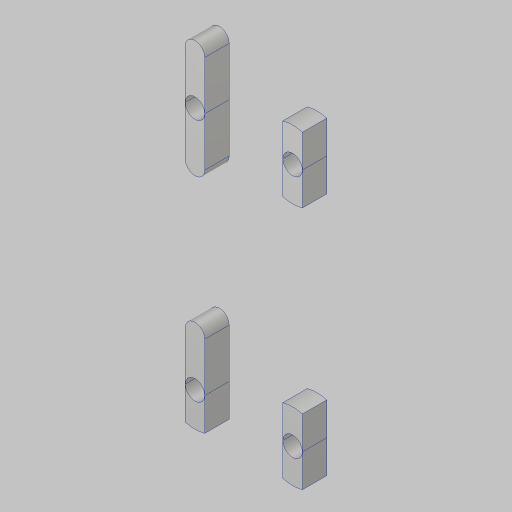
# Autodesk Inventor part: CL8-GB-001
Saved by Autodesk Inventor 2023.5 (Build 275446000, 446)
## iProperties
Created: 2025-03-18
Part Number: CL8-GB-001
Material: Aluminum 6061
Document SubType Name: Modeling
Designer: slick
Density: 2.7 g/cm^3
Appearance: Aluminum - Flat
Mass: 157.99 g
Surface Area: 311.753 cm^2
Volume: 58.5147 cm^3
Author: slick
Autodesk Inventor part; units mm, degrees
ref_plane "YZ Plane" through (0, 0, 0) normal (1, 0, 0) x (0, 1, 0)
ref_plane "XZ Plane" through (0, 0, 0) normal (0, 1, 0) x (-1, 0, 0)
ref_plane "XY Plane" through (0, 0, 0) normal (0, 0, 1) x (1, 0, 0)
sketch "Sketch1" plane through (0, 0, 0) normal (0, 0, 1) x (1, 0, 0)
  line L0 (0, 0) -> (-50.8, 0) construction
  line L1 (-50.8, 0) -> (-50.8, 381) construction
  line L2 (-50.8, 381) -> (0, 381) construction
  line L3 (0, 381) -> (0, 0) construction
  circle A0 centre (-50.8, 431.8) radius 11.1125 construction
  line L4 (-50.8, 353.7099) -> (-298.4703, 0) construction
  line L5 (-298.4703, 0) -> (-267.4626, 0) construction
  line L6 (-267.4626, 0) -> (-50.8, 309.4263) construction
  dimension "d0" = 50.8
  dimension "d1" = 381
  dimension "d2" = 22.225
  dimension "d3" = 431.8
  dimension "d4" = 50.8
  dimension "d5" = 431.8
  dimension "d6" = 25.4
  dimension "d7" = 35
  constraints: 14 end point, 3 parallel, 2 horizontal, 2 point on line, 1 centre point, 1 collinear, 1 perpendicular
  measures "d0" distance of L1.end L2.end
  measures "d1" distance of L0.end L1.end
  measures "d2" diameter of A0
  measures "d3" distance from line of L0 A0.centre
  measures "d4" distance from line of L3 A0.centre
  measures "d5" distance of L4.start L4.end
  measures "d6" distance between parallel lines of L6 L4
  measures "d7" angle of L1 L4
sketch "Sketch2" plane through (0, 0, 0) normal (0, 0, 1) x (1, 0, 0)
  line L0 (-267.4626, 0) -> (-50.8, 309.4263) construction
  line L1 (-50.8, 353.7099) -> (-298.4703, 0) construction
  line L2 (-50.8, 0) -> (-50.8, 381) construction
  line L3 (0, 381) -> (0, 0) construction
  line L4 (-50.8, 381) -> (0, 381) construction
  circle A0 centre (-50.8, 431.8) radius 11.1125 construction
  line L5 (0, 0) -> (-50.8, 0) construction
  line L6 (-298.4703, 0) -> (-267.4626, 0) construction
  circle A1 centre (-88.9, 38.1) radius 30.48 construction
  circle A2 centre (-88.9, 38.1) radius 6.35 construction
  circle A3 centre (-99.4866, 89.0824) radius 45.72 construction
  circle A4 centre (-99.4866, 89.0824) radius 11.43 construction
  circle A5 centre (-157.9039, 88.5265) radius 46.99 construction
  circle A6 centre (-157.9039, 88.5265) radius 12.7 construction
  circle A7 centre (-140.3916, 141.5914) radius 43.18 construction
  circle A8 centre (-99.4866, 89.0824) radius 14.2875
  circle A9 centre (-157.9039, 88.5265) radius 14.2875
  circle A10 centre (-140.3916, 141.5914) radius 14.2875
  circle A11 centre (-50.8, 431.8) radius 54.5719 construction
  line L7 (-50.8, 177.8) -> (0, 177.8)
  circle A12 centre (-140.3916, 141.5914) radius 20.6375 construction
  circle A13 centre (-157.9039, 88.5265) radius 20.6375 construction
  circle A14 centre (-99.4866, 89.0824) radius 20.6375 construction
  circle A15 centre (-88.9, 38.1) radius 25.4 construction
  line L8 (-50.8, 177.8) -> (-143.8598, 161.9354)
  line L9 (-74.6041, 11.1805) -> (0, 50.8)
  line L10 (0, 177.8) -> (0, 50.8)
  arc A16 (-143.8598, 161.9354) -> (-158.347, 131.4176) centre (-140.3916, 141.5914) ccw
  arc A17 (-117.4357, 99.2675) -> (-118.6127, 96.8346) centre (-99.4866, 89.0824) ccw
  arc A18 (-118.8586, 43.7135) -> (-74.6041, 11.1805) centre (-88.9, 38.1) ccw
  line L11 (-38.1, 152.4) -> (-38.1, 127) construction
  line L12 (-40.6527, 152.4) -> (-40.6527, 127)
  line L13 (-35.5473, 127) -> (-35.5473, 152.4)
  arc A19 (-35.5473, 152.4) -> (-40.6527, 152.4) centre (-38.1, 152.4) ccw
  arc A20 (-40.6527, 127) -> (-35.5473, 127) centre (-38.1, 127) ccw
  line L14 (-12.7, 152.4) -> (-12.7, 127) construction
  line L15 (-15.2527, 152.4) -> (-15.2527, 127)
  line L16 (-10.1473, 127) -> (-10.1473, 152.4)
  arc A21 (-10.1473, 152.4) -> (-15.2527, 152.4) centre (-12.7, 152.4) ccw
  arc A22 (-15.2527, 127) -> (-10.1473, 127) centre (-12.7, 127) ccw
  line L17 (-38.1, 139.7) -> (-12.7, 139.7) construction
  line L18 (-38.1, 88.9) -> (-38.1, 63.5) construction
  line L19 (-40.6527, 88.9) -> (-40.6527, 63.5)
  line L20 (-35.5473, 63.5) -> (-35.5473, 88.9)
  arc A23 (-35.5473, 88.9) -> (-40.6527, 88.9) centre (-38.1, 88.9) ccw
  arc A24 (-40.6527, 63.5) -> (-35.5473, 63.5) centre (-38.1, 63.5) ccw
  line L21 (-12.7, 88.9) -> (-12.7, 63.5) construction
  line L22 (-15.2527, 88.9) -> (-15.2527, 63.5)
  line L23 (-10.1473, 63.5) -> (-10.1473, 88.9)
  arc A25 (-10.1473, 88.9) -> (-15.2527, 88.9) centre (-12.7, 88.9) ccw
  arc A26 (-15.2527, 63.5) -> (-10.1473, 63.5) centre (-12.7, 63.5) ccw
  line L24 (-38.1, 76.2) -> (-12.7, 76.2) construction
  circle A27 centre (-88.9, 38.1) radius 10.795
  point P0 (-88.9, 63.5)
  point P1 (-110.897, 50.8)
  point P2 (-110.897, 25.4)
  point P3 (-88.9, 12.7)
  point P4 (-66.903, 25.4)
  point P5 (-66.903, 50.8)
  point P6 (-25.4, 139.7)
  point P7 (-25.4, 177.8)
  point P8 (-25.4, 76.2)
  point P9 (-38.1, 168.275)
  point P10 (-12.7, 168.275)
  dimension "d25" = 50.8
  dimension "d8" = 60.96
  dimension "d9" = 12.7
  dimension "d10" = 91.44
  dimension "d11" = 38.1
  dimension "d12" = 38.1
  dimension "d13" = 22.86
  dimension "d14" = 93.98
  dimension "d15" = 25.4
  dimension "d16" = 86.36
  dimension "d22" = 28.575
  dimension "d23" = 109.1438
  dimension "d24" = 6.35
  dimension "d28" = 360
  dimension "d30" = 177.8
  dimension "d31" = 50.8
  dimension "d32" = 5.1054
  dimension "d33" = 25.4
  dimension "d34" = 38.1
  dimension "d35" = 25.4
  dimension "d36" = 5.1054
  dimension "d37" = 25.4
  dimension "d38" = 25.4
  dimension "d39" = 63.5
  dimension "d42" = 21.59
  dimension "d50" = 9.525
  constraints: 44 end point, 28 point on circle, 26 centre point, 21 tangent, 18 coincident, 7 midpoint, 6 equal radius, 6 parallel, 6 vertical alignment, 5 horizontal alignment, 3 horizontal, 3 point on line, 2 vertical, 1 collinear, 9 other
  measures "d8" diameter of A1
  measures "d9" diameter of A2
  measures "d10" diameter of A3
  measures "d11" distance from line of L5 A1.centre
  measures "d12" distance from line of L2 A1.centre
  measures "d13" diameter of A4
  measures "d14" diameter of A5
  measures "d15" diameter of A6
  measures "d16" diameter of A7
  measures "d22" diameter of A8
  measures "d23" diameter of A11
  measures "d24" radial gap between concentric circles of A10 A12
  measures "d30" distance between parallel lines of L5 L7
  measures "d31" distance from line of L5 L9.end
  measures "d32" diameter of A20
  measures "d33" distance of L11.start L11.end
  measures "d34" distance from line of L7 L17.start
  measures "d35" distance of L17.start L17.end
  measures "d36" diameter of A24
  measures "d37" distance of L18.start L18.end
  measures "d38" distance of L24.start L24.end
  measures "d39" distance between parallel lines of L17 L24
  measures "d42" diameter of A27
  measures "d50" distance from line of L7 point (-38.1, 168.275)
extrude "Extrusion1" add sketch "Sketch2" along normal blind 6.35 contours A19 L13 A20 L12 | A21 L16 A22 L15 | A23 L20 A24 L19 | A25 L23 A26 L22
hole "Hole1" at (-88.9, 63.5, 0) at (-110.897, 50.8, 0) at (-110.897, 25.4, 0) at (-88.9, 12.7, 0) at (-66.903, 25.4, 0) at (-66.903, 50.8, 0) at (-38.1, 139.7, 0) at (-12.7, 139.7, 0) at (-38.1, 76.2, 0) at (-12.7, 76.2, 0) direction (0, 0, 1) diameter 5.1054 end through all clearance for "Flat Head Machine Screw (82)" size "#10" standard "Ansi Unified Screw Threads"
fillet "Fillet1" [suppressed]
hole "Hole2" at (-38.1, 168.275, 0) at (-12.7, 168.275, 0) direction (0, 0, 1) diameter 3.9624 end through all thread size "10-32 UNF" class "2B" standard "ANSI Unified Screw Threads"
sketch "Sketch4" plane through (0, 0, 6.35) normal (0, 0, 1) x (1, 0, 0)
  arc A0 (-35.5473, 76.2) -> (-40.6527, 76.2) centre (-38.1, 76.2) ccw construction
  arc A1 (-35.5473, 139.7) -> (-40.6527, 139.7) centre (-38.1, 139.7) ccw construction
  arc A2 (-10.1473, 139.7) -> (-15.2527, 139.7) centre (-12.7, 139.7) ccw construction
  arc A3 (-10.1473, 76.2) -> (-15.2527, 76.2) centre (-12.7, 76.2) ccw construction
  line L0 (-35.5473, 139.7) -> (-35.5473, 152.4) projected
  arc A4 (-35.5473, 152.4) -> (-40.6527, 152.4) centre (-38.1, 152.4) ccw projected
  line L1 (-40.6527, 152.4) -> (-40.6527, 139.7) projected
  arc A5 (-40.6527, 139.7) -> (-35.5473, 139.7) centre (-38.1, 139.7) ccw projected
  line L2 (-40.6527, 139.7) -> (-40.6527, 127) projected
  arc A6 (-40.6527, 127) -> (-35.5473, 127) centre (-38.1, 127) ccw projected
  line L3 (-35.5473, 127) -> (-35.5473, 139.7) projected
  line L4 (-35.5473, 76.2) -> (-35.5473, 88.9) projected
  arc A7 (-35.5473, 88.9) -> (-40.6527, 88.9) centre (-38.1, 88.9) ccw projected
  line L5 (-40.6527, 88.9) -> (-40.6527, 76.2) projected
  arc A8 (-40.6527, 76.2) -> (-35.5473, 76.2) centre (-38.1, 76.2) ccw projected
  line L6 (-40.6527, 76.2) -> (-40.6527, 63.5) projected
  arc A9 (-40.6527, 63.5) -> (-35.5473, 63.5) centre (-38.1, 63.5) ccw projected
  line L7 (-35.5473, 63.5) -> (-35.5473, 76.2) projected
  line L8 (-10.1473, 139.7) -> (-10.1473, 152.4) projected
  arc A10 (-10.1473, 152.4) -> (-15.2527, 152.4) centre (-12.7, 152.4) ccw projected
  line L9 (-15.2527, 152.4) -> (-15.2527, 139.7) projected
  arc A11 (-15.2527, 139.7) -> (-10.1473, 139.7) centre (-12.7, 139.7) ccw projected
  line L10 (-15.2527, 139.7) -> (-15.2527, 127) projected
  arc A12 (-15.2527, 127) -> (-10.1473, 127) centre (-12.7, 127) ccw projected
  line L11 (-10.1473, 127) -> (-10.1473, 139.7) projected
  line L12 (-10.1473, 76.2) -> (-10.1473, 88.9) projected
  arc A13 (-10.1473, 88.9) -> (-15.2527, 88.9) centre (-12.7, 88.9) ccw projected
  line L13 (-15.2527, 88.9) -> (-15.2527, 76.2) projected
  arc A14 (-15.2527, 76.2) -> (-10.1473, 76.2) centre (-12.7, 76.2) ccw projected
  line L14 (-15.2527, 76.2) -> (-15.2527, 63.5) projected
  arc A15 (-15.2527, 63.5) -> (-10.1473, 63.5) centre (-12.7, 63.5) ccw projected
  line L15 (-10.1473, 63.5) -> (-10.1473, 76.2) projected
  point P0 (0, 0)
  point P1 (-64.4644, 155.575)
hole "Hole3" at (-64.4644, 155.575, 6.35) direction (0, 0, -1) diameter 3.9624 end through all thread size "10-32 UNF" class "2B" standard "ANSI Unified Screw Threads"
sketch "Sketch3" plane through (0, 0, 6.35) normal (0, 0, 1) x (1, 0, 0)
  arc A0 (-35.5473, 76.2) -> (-40.6527, 76.2) centre (-38.1, 76.2) ccw construction
  arc A1 (-35.5473, 139.7) -> (-40.6527, 139.7) centre (-38.1, 139.7) ccw construction
  arc A2 (-10.1473, 139.7) -> (-15.2527, 139.7) centre (-12.7, 139.7) ccw construction
  arc A3 (-10.1473, 76.2) -> (-15.2527, 76.2) centre (-12.7, 76.2) ccw construction
  circle A4 centre (-101.6, 129.9906) radius 20.6375 construction
  arc A5 (-136.4593, 83.8492) -> (-111.3998, 184.5895) centre (-275.3417, 171.8837) ccw construction
  arc A6 (-88.8183, 197.2966) -> (-111.3998, 184.5895) centre (-97.155, 185.6935) ccw construction
  line L0 (-61.7546, 177.8517) -> (-94.3408, 201.2645) construction
  arc A7 (-56.2321, 173.8838) -> (-48.6735, 171.45) centre (-48.6735, 184.404) ccw construction
  line L1 (-48.6735, 171.45) -> (-6.604, 171.45) construction
  arc A8 (-6.35, 171.196) -> (-6.604, 171.45) centre (-6.604, 171.196) ccw
  line L2 (-6.35, 171.196) -> (-6.35, 54.7703) construction
  arc A9 (-6.4849, 54.546) -> (-6.35, 54.7703) centre (-6.604, 54.7703) ccw
  line L3 (-6.4849, 54.546) -> (-77.5824, 16.7888) construction
  arc A10 (-109.3468, 25.2865) -> (-77.5824, 16.7888) centre (-88.9, 38.1) ccw construction
  line L4 (-109.3468, 25.2865) -> (-136.4985, 68.613) construction
  arc A11 (-136.4593, 83.8492) -> (-136.4985, 68.613) centre (-124.3919, 76.2) ccw construction
  circle A12 centre (-97.155, 185.6935) radius 20.6375 construction
  circle A13 centre (-124.3919, 76.2) radius 20.6375 construction
  circle A14 centre (-38.1, 139.7) radius 8.9027 construction
  arc A15 (-10.1473, 139.7) -> (-15.2527, 139.7) centre (-12.7, 139.7) ccw construction
  circle A16 centre (-12.7, 139.7) radius 8.9027 construction
  arc A17 (-10.1473, 76.2) -> (-15.2527, 76.2) centre (-12.7, 76.2) ccw construction
  circle A18 centre (-12.7, 76.2) radius 8.9027 construction
  arc A19 (-35.5473, 76.2) -> (-40.6527, 76.2) centre (-38.1, 76.2) ccw construction
  circle A20 centre (-38.1, 76.2) radius 8.9027 construction
  circle A21 centre (-66.903, 50.8) radius 2.5527 construction
  circle A22 centre (-66.903, 50.8) radius 8.9027 construction
  circle A23 centre (-88.9, 63.5) radius 8.9027 construction
  circle A24 centre (-38.1, 168.275) radius 1.9812 construction
  circle A25 centre (-38.1, 168.275) radius 8.9027 construction
  circle A26 centre (-12.7, 168.275) radius 1.9812 construction
  circle A27 centre (-12.7, 168.275) radius 8.9027 construction
  line L5 (-101.6, 129.9906) -> (-38.1, 139.7) construction
  circle A28 centre (-88.9, 63.5) radius 2.5527 construction
  line L6 (-124.3919, 76.2) -> (-88.9, 63.5) construction
  line L7 (-88.9, 63.5) -> (-66.903, 50.8) construction
  line L8 (-66.903, 50.8) -> (-38.1, 76.2) construction
  arc A29 (-35.5473, 139.7) -> (-40.6527, 139.7) centre (-38.1, 139.7) ccw construction
  line L9 (-38.1, 139.7) -> (-38.1, 76.2) construction
  line L10 (-102.0799, 133.1291) -> (-38.5799, 142.8385) construction
  line L11 (-101.1201, 126.852) -> (-37.6201, 136.5615) construction
  line L12 (-41.275, 139.7) -> (-41.275, 77.6333) construction
  line L13 (-41.275, 77.6333) -> (-67.2915, 54.6905) construction
  line L14 (-67.2915, 54.6905) -> (-87.5606, 66.3929) construction
  line L15 (-87.5606, 66.3929) -> (-123.3222, 79.1894) construction
  line L16 (-34.925, 141.1333) -> (-34.925, 74.7667) construction
  line L17 (-34.925, 74.7667) -> (-66.5144, 46.9095) construction
  line L18 (-66.5144, 46.9095) -> (-90.2394, 60.6071) construction
  line L19 (-90.2394, 60.6071) -> (-125.4616, 73.2106) construction
  line L20 (-38.1, 139.7) -> (-38.1, 168.275) construction
  line L21 (-34.925, 107.95) -> (-6.35, 107.95) construction
  line L22 (-34.925, 111.125) -> (-6.35, 111.125) construction
  line L23 (-34.925, 104.775) -> (-6.35, 104.775) construction
  line L24 (-34.925, 139.7) -> (-34.925, 168.275) construction
  line L25 (-41.275, 139.7) -> (-41.275, 168.275) construction
  line L26 (-76.7242, 188.6072) -> (-56.2321, 173.8838)
  line L27 (-48.6735, 171.45) -> (-46.4173, 171.45)
  line L28 (-29.7827, 171.45) -> (-21.0173, 171.45)
  line L29 (-6.35, 162.0352) -> (-6.35, 145.9398)
  line L30 (-6.35, 133.4602) -> (-6.35, 111.125)
  line L31 (-6.35, 111.125) -> (-34.925, 111.125)
  line L32 (-34.925, 111.125) -> (-34.925, 131.3827)
  line L33 (-34.925, 148.0173) -> (-34.925, 159.9577)
  line L34 (-41.275, 159.9577) -> (-41.275, 148.0173)
  line L35 (-6.35, 104.775) -> (-34.925, 104.775)
  line L36 (-34.925, 104.775) -> (-34.925, 84.5173)
  line L37 (-6.35, 104.775) -> (-6.35, 82.4398)
  line L38 (-6.35, 69.9602) -> (-6.35, 54.7703)
  line L39 (-6.4849, 54.546) -> (-55.1495, 28.702)
  line L40 (-58.5648, 53.9198) -> (-42.2382, 68.3175)
  line L41 (-72.5184, 57.7083) -> (-80.1095, 62.091)
  line L42 (-62.7648, 58.6825) -> (-46.4381, 73.0802)
  line L43 (-95.6614, 69.2915) -> (-104.1226, 72.3192)
  line L44 (-41.275, 84.5173) -> (-41.275, 131.3827)
  line L45 (-45.8418, 135.3043) -> (-80.9626, 129.9342)
  line L46 (-81.9224, 136.2113) -> (-46.8016, 141.5814)
  arc A30 (-110.9157, 170.3133) -> (-76.7242, 188.6072) centre (-97.155, 185.6935) ccw
  arc A31 (-81.9224, 136.2113) -> (-112.7474, 147.3584) centre (-101.6, 129.9906) ccw
  arc A32 (-41.275, 148.0173) -> (-46.8016, 141.5814) centre (-38.1, 139.7) ccw
  arc A33 (-46.4173, 171.45) -> (-41.275, 159.9577) centre (-38.1, 168.275) ccw
  arc A34 (-56.2321, 173.8838) -> (-48.6735, 171.45) centre (-48.6735, 184.404) ccw
  arc A35 (-21.0173, 171.45) -> (-6.35, 162.0352) centre (-12.7, 168.275) ccw
  arc A36 (-6.35, 145.9398) -> (-6.35, 133.4602) centre (-12.7, 139.7) ccw
  arc A37 (-34.925, 131.3827) -> (-34.925, 148.0173) centre (-38.1, 139.7) ccw
  arc A38 (-119.4378, 119.6117) -> (-80.9626, 129.9342) centre (-101.6, 129.9906) ccw
  arc A39 (-104.1226, 72.3192) -> (-129.3429, 96.2348) centre (-124.3919, 76.2) ccw
  arc A40 (-80.1095, 62.091) -> (-95.6614, 69.2915) centre (-88.9, 63.5) ccw
  arc A41 (-62.7648, 58.6825) -> (-72.5184, 57.7083) centre (-66.903, 50.8) ccw
  arc A42 (-41.275, 84.5173) -> (-46.4381, 73.0802) centre (-38.1, 76.2) ccw
  arc A43 (-6.35, 82.4398) -> (-6.35, 69.9602) centre (-12.7, 76.2) ccw
  arc A44 (-62.7274, 42.9373) -> (-58.5648, 53.9198) centre (-66.903, 50.8) ccw
  arc A45 (-42.2382, 68.3175) -> (-34.925, 84.5173) centre (-38.1, 76.2) ccw
  arc A46 (-112.7474, 147.3584) -> (-110.9157, 170.3133) centre (-275.3417, 171.8837) ccw
  arc A47 (-129.3429, 96.2348) -> (-119.4378, 119.6117) centre (-275.3417, 171.8837) ccw
  arc A48 (-34.925, 159.9577) -> (-29.7827, 171.45) centre (-38.1, 168.275) ccw
  arc A49 (-45.8418, 135.3043) -> (-41.275, 131.3827) centre (-38.1, 139.7) ccw
  line L47 (-62.7134, 42.945) -> (-55.1495, 28.702)
  arc A50 (-128.5905, 55.9941) -> (-104.1226, 72.3192) centre (-124.3919, 76.2) ccw
  arc A51 (-129.3429, 96.2348) -> (-128.5905, 55.9941) centre (-124.3919, 76.2) ccw
  circle A52 centre (-64.4644, 155.575) radius 1.9812 construction
  circle A53 centre (-64.4644, 155.575) radius 8.9027 construction
  line L48 (-97.155, 185.6935) -> (-64.4644, 155.575) construction
  line L49 (-64.4644, 155.575) -> (-38.1, 168.275) construction
  line L50 (-95.0037, 188.0285) -> (-63.8992, 159.3714) construction
  line L51 (-63.8992, 159.3714) -> (-39.4779, 171.1354) construction
  line L52 (-36.7221, 165.4146) -> (-65.0295, 151.7786) construction
  line L53 (-65.0295, 151.7786) -> (-99.3063, 183.3585) construction
  line L54 (-84.3092, 169.5413) -> (-72.7326, 158.8756)
  line L55 (-80.0066, 174.2114) -> (-68.43, 163.5457)
  line L56 (-58.349, 162.045) -> (-46.9711, 167.5259)
  line L57 (-44.2153, 161.805) -> (-55.5932, 156.3241)
  arc A54 (-72.7326, 158.8756) -> (-55.5932, 156.3241) centre (-64.4644, 155.575) ccw
  arc A55 (-58.349, 162.045) -> (-68.43, 163.5457) centre (-64.4644, 155.575) ccw
  line L58 (-35.5473, 139.7) -> (-35.5473, 152.4) projected
  arc A56 (-35.5473, 152.4) -> (-40.6527, 152.4) centre (-38.1, 152.4) ccw projected
  line L59 (-40.6527, 152.4) -> (-40.6527, 139.7) projected
  arc A57 (-40.6527, 139.7) -> (-35.5473, 139.7) centre (-38.1, 139.7) ccw projected
  line L60 (-40.6527, 139.7) -> (-40.6527, 127) projected
  arc A58 (-40.6527, 127) -> (-35.5473, 127) centre (-38.1, 127) ccw projected
  line L61 (-35.5473, 127) -> (-35.5473, 139.7) projected
  line L62 (-35.5473, 76.2) -> (-35.5473, 88.9) projected
  arc A59 (-35.5473, 88.9) -> (-40.6527, 88.9) centre (-38.1, 88.9) ccw projected
  line L63 (-40.6527, 88.9) -> (-40.6527, 76.2) projected
  arc A60 (-40.6527, 76.2) -> (-35.5473, 76.2) centre (-38.1, 76.2) ccw projected
  line L64 (-40.6527, 76.2) -> (-40.6527, 63.5) projected
  arc A61 (-40.6527, 63.5) -> (-35.5473, 63.5) centre (-38.1, 63.5) ccw projected
  line L65 (-35.5473, 63.5) -> (-35.5473, 76.2) projected
  line L66 (-10.1473, 139.7) -> (-10.1473, 152.4) projected
  arc A62 (-10.1473, 152.4) -> (-15.2527, 152.4) centre (-12.7, 152.4) ccw projected
  line L67 (-15.2527, 152.4) -> (-15.2527, 139.7) projected
  arc A63 (-15.2527, 139.7) -> (-10.1473, 139.7) centre (-12.7, 139.7) ccw projected
  line L68 (-15.2527, 139.7) -> (-15.2527, 127) projected
  arc A64 (-15.2527, 127) -> (-10.1473, 127) centre (-12.7, 127) ccw projected
  line L69 (-10.1473, 127) -> (-10.1473, 139.7) projected
  line L70 (-10.1473, 76.2) -> (-10.1473, 88.9) projected
  arc A65 (-10.1473, 88.9) -> (-15.2527, 88.9) centre (-12.7, 88.9) ccw projected
  line L71 (-15.2527, 88.9) -> (-15.2527, 76.2) projected
  arc A66 (-15.2527, 76.2) -> (-10.1473, 76.2) centre (-12.7, 76.2) ccw projected
  line L72 (-15.2527, 76.2) -> (-15.2527, 63.5) projected
  arc A67 (-15.2527, 63.5) -> (-10.1473, 63.5) centre (-12.7, 63.5) ccw projected
  line L73 (-10.1473, 63.5) -> (-10.1473, 76.2) projected
  point P0 (0, 0)
  point P1 (-62.7133, 42.9448)
  dimension "d65" = 6.35
  dimension "d66" = 3.175
  dimension "d67" = 3.175
  dimension "d68" = 3.175
  dimension "d69" = 3.175
  dimension "d70" = 63.5
  dimension "d71" = 3.175
  dimension "d72" = 3.175
  dimension "d73" = 3.175
  dimension "d74" = 3.175
  dimension "d75" = 25.4
  dimension "d90" = 3.175
  dimension "d91" = 3.175
  constraints: 116 end point, 108 point on circle, 43 centre point, 39 point on line, 31 coincident, 10 equal radius, 7 collinear, 6 parallel, 2 horizontal, 2 vertical, 1 midpoint, 1 perpendicular, 1 tangent, 8 other
  measures "d65" radial gap between concentric circles of A1 A14
  measures "d66" distance between parallel lines of L5 L10
  measures "d67" distance between parallel lines of L5 L11
  measures "d68" distance between parallel lines of L9 L12
  measures "d69" distance between parallel lines of L9 L16
  measures "d70" distance between parallel lines of L1 L21
  measures "d71" distance between parallel lines of L21 L22
  measures "d72" distance between parallel lines of L21 L23
  measures "d73" distance between parallel lines of L20 L24
  measures "d74" distance between parallel lines of L20 L25
  measures "d75" distance from line of A10.centre L47
  measures "d90" distance between parallel lines of L48 L50
  measures "d91" distance between parallel lines of L49 L52
extrude "Extrusion2" cut sketch "Sketch3" against normal through all contours L39 L47 A44 L40 A45 L64 A61 L65 L36 L35 L37 A43 L70 A65 L71 L72 A67 L73 L38 A9 | L73 A67 L72 A43 | L71 A65 L70 A43 | A45 L65 A61 L64 | L26 A34 L27 A33 L56 A55 L55 A30 | L55 A55 L56 A33 L57 A54 L54 A30 | L54 A54 L57 A33 L34 A32 L46 A31 A46 A30 | L28 A35 L29 A36 L66 A62 L67 L68 A64 L69 L30 L31 L32 A37 L33 A48 | A36 L67 A62 L66 | A36 L69 A64 L68 | L41 A40 L43 A39 A47 A38 L45 A49 L44 A42 L42 A41
fillet "Fillet2" [suppressed]
body "Solid1"
